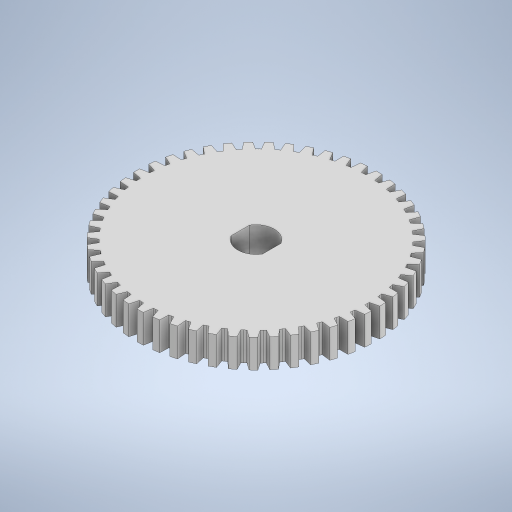
# Autodesk Inventor part: Tandwiel
Saved by Autodesk Inventor 2023.2 (Build 272271030, 271C)
## iProperties
Created: 2023-03-15
Part Number: Tandwiel
Material: Generic
Document SubType Name: Modeling
Designer: daanj
Density: 1 g/cm^3
Appearance: Default
Author: daanj
Autodesk Inventor part; units mm, degrees
ref_plane "YZ Plane" through (0, 0, 0) normal (1, 0, 0) x (0, 1, 0)
ref_plane "XZ Plane" through (0, 0, 0) normal (0, 1, 0) x (-1, 0, 0)
ref_plane "XY Plane" through (0, 0, 0) normal (0, 0, 1) x (1, 0, 0)
sketch "Sketch1" plane through (0, 0, 0) normal (0, 1, 0) x (-1, 0, 0)
  line L0 (0, 0) -> (25.1689, -1.5524) construction
  line L1 (0, 0) -> (25.1122, 1.5489) construction
  line L2 (0, 0) -> (25.4925, 0) construction
  line L3 (19.4825, 0.8259) -> (20.993, 0.5434)
  line L4 (20.993, -0.5434) -> (19.4825, -0.8259)
  line L5 (19.463, 1.2004) -> (19.4825, 0.8259)
  line L6 (19.4825, -0.8259) -> (19.463, -1.2004)
  arc A0 (20.993, -0.5434) -> (20.993, 0.5434) centre (0, 0) ccw
  line L7 (19.168, 3.5831) -> (19.2333, 3.2138)
  line L8 (19.2333, 3.2138) -> (20.7671, 3.119)
  arc A1 (20.9006, 2.0405) -> (20.7671, 3.119) centre (0, 0) ccw
  line L9 (20.9006, 2.0405) -> (19.4363, 1.5745)
  line L10 (19.4363, 1.5745) -> (19.463, 1.2004)
  line L11 (18.5824, 5.9115) -> (18.6926, 5.553)
  line L12 (18.6926, 5.553) -> (20.2264, 5.6474)
  arc A2 (20.4915, 4.5935) -> (20.2264, 5.6474) centre (0, 0) ccw
  line L13 (20.4915, 4.5935) -> (19.0955, 3.9511)
  line L14 (19.0955, 3.9511) -> (19.168, 3.5831)
  line L15 (17.7151, 8.1502) -> (17.8685, 7.808)
  line L16 (17.8685, 7.808) -> (19.3791, 8.0902)
  arc A3 (19.7717, 7.0769) -> (19.3791, 8.0902) centre (0, 0) ccw
  line L17 (19.7717, 7.0769) -> (18.4653, 6.2677)
  line L18 (18.4653, 6.2677) -> (18.5824, 5.9115)
  line L19 (16.5792, 10.2654) -> (16.7736, 9.9447)
  line L20 (16.7736, 9.9447) -> (18.238, 10.4104)
  arc A4 (18.7521, 9.4529) -> (18.238, 10.4104) centre (0, 0) ccw
  line L21 (18.7521, 9.4529) -> (17.5551, 8.4894)
  line L22 (17.5551, 8.4894) -> (17.7151, 8.1502)
  line L23 (15.1921, 12.225) -> (15.4244, 11.9306)
  line L24 (15.4244, 11.9306) -> (16.8204, 12.5727)
  arc A5 (17.4483, 11.6857) -> (16.8204, 12.5727) centre (0, 0) ccw
  line L25 (17.4483, 11.6857) -> (16.3788, 10.5824)
  line L26 (16.3788, 10.5824) -> (16.5792, 10.2654)
  line L27 (13.5746, 13.9993) -> (13.8413, 13.7356)
  line L28 (13.8413, 13.7356) -> (15.1479, 14.5444)
  arc A6 (15.8801, 13.7413) -> (15.1479, 14.5444) centre (0, 0) ccw
  line L29 (15.8801, 13.7413) -> (14.9542, 12.5149)
  line L30 (14.9542, 12.5149) -> (15.1921, 12.225)
  line L31 (11.7514, 15.5613) -> (12.0485, 15.3325)
  line L32 (12.0485, 15.3325) -> (13.2458, 16.2957)
  arc A7 (14.0711, 15.5886) -> (13.2458, 16.2957) centre (0, 0) ccw
  line L33 (14.0711, 15.5886) -> (13.3029, 14.2577)
  line L34 (13.3029, 14.2577) -> (13.5746, 13.9993)
  line L35 (9.75, 16.8875) -> (10.073, 16.6969)
  line L36 (10.073, 16.6969) -> (11.1428, 17.7999)
  arc A8 (12.0487, 17.1996) -> (11.1428, 17.7999) centre (0, 0) ccw
  line L37 (12.0487, 17.1996) -> (11.4499, 15.7844)
  line L38 (11.4499, 15.7844) -> (11.7514, 15.5613)
  line L39 (7.6008, 17.9577) -> (7.9448, 17.8082)
  line L40 (7.9448, 17.8082) -> (8.871, 19.0343)
  arc A9 (9.8438, 18.5499) -> (8.871, 19.0343) centre (0, 0) ccw
  line L41 (9.8438, 18.5499) -> (9.4234, 17.0719)
  line L42 (9.4234, 17.0719) -> (9.75, 16.8875)
  line L43 (5.3364, 18.7556) -> (5.6961, 18.6495)
  line L44 (5.6961, 18.6495) -> (6.4646, 19.9802)
  arc A10 (7.4896, 19.619) -> (6.4646, 19.9802) centre (0, 0) ccw
  line L45 (7.4896, 19.619) -> (7.2541, 18.1005)
  line L46 (7.2541, 18.1005) -> (7.6008, 17.9577)
  line L47 (2.9911, 19.2692) -> (3.3611, 19.2081)
  line L48 (3.3611, 19.2081) -> (3.9603, 20.6232)
  arc A11 (5.0219, 20.3907) -> (3.9603, 20.6232) centre (0, 0) ccw
  line L49 (5.0219, 20.3907) -> (4.9748, 18.8548)
  line L50 (4.9748, 18.8548) -> (5.3364, 18.7556)
  line L51 (0.6005, 19.4908) -> (0.9752, 19.4756)
  line L52 (0.9752, 19.4756) -> (1.3959, 20.9536)
  arc A12 (2.478, 20.8533) -> (1.3959, 20.9536) centre (0, 0) ccw
  line L53 (2.478, 20.8533) -> (2.62, 19.3232)
  line L54 (2.62, 19.3232) -> (2.9911, 19.2692)
  line L55 (-1.7992, 19.4168) -> (-1.4255, 19.4478)
  line L56 (-1.4255, 19.4478) -> (-1.1896, 20.9663)
  arc A13 (-0.1034, 20.9997) -> (-1.1896, 20.9663) centre (0, 0) ccw
  line L57 (-0.1034, 20.9997) -> (0.2256, 19.4987)
  line L58 (0.2256, 19.4987) -> (0.6005, 19.4908)
  line L59 (-4.1717, 19.0485) -> (-3.8046, 19.1252)
  line L60 (-3.8046, 19.1252) -> (-3.7571, 20.6612)
  arc A14 (-2.6832, 20.8279) -> (-3.7571, 20.6612) centre (0, 0) ccw
  line L61 (-2.6832, 20.8279) -> (-2.1723, 19.3786)
  line L62 (-2.1723, 19.3786) -> (-1.7992, 19.4168)
  line L63 (-6.4809, 18.3915) -> (-6.126, 18.5127)
  line L64 (-6.126, 18.5127) -> (-6.2676, 20.0429)
  arc A15 (-5.2224, 20.3403) -> (-6.2676, 20.0429) centre (0, 0) ccw
  line L65 (-5.2224, 20.3403) -> (-4.5372, 18.9648)
  line L66 (-4.5372, 18.9648) -> (-4.1717, 19.0485)
  line L67 (-8.6919, 17.4557) -> (-8.3546, 17.6196)
  line L68 (-8.3546, 17.6196) -> (-8.6832, 19.1207)
  arc A16 (-7.6824, 19.5443) -> (-8.6832, 19.1207) centre (0, 0) ccw
  line L69 (-7.6824, 19.5443) -> (-6.8334, 18.2635)
  line L70 (-6.8334, 18.2635) -> (-6.4809, 18.3915)
  line L71 (-10.7711, 16.2552) -> (-10.4565, 16.4594)
  line L72 (-10.4565, 16.4594) -> (-10.9671, 17.9088)
  arc A17 (-10.0259, 18.4521) -> (-10.9671, 17.9088) centre (0, 0) ccw
  line L73 (-10.0259, 18.4521) -> (-9.026, 17.2853)
  line L74 (-9.026, 17.2853) -> (-8.6919, 17.4557)
  line L75 (-12.6871, 14.8084) -> (-12.3999, 15.0496)
  line L76 (-12.3999, 15.0496) -> (-13.0847, 16.4253)
  arc A18 (-12.2175, 17.0802) -> (-13.0847, 16.4253) centre (0, 0) ccw
  line L77 (-12.2175, 17.0802) -> (-11.0817, 16.0451)
  line L78 (-11.0817, 16.0451) -> (-10.7711, 16.2552)
  line L79 (-14.4107, 13.1371) -> (-14.1554, 13.4118)
  line L80 (-14.1554, 13.4118) -> (-15.004, 14.6928)
  arc A19 (-14.2238, 15.4494) -> (-15.004, 14.6928) centre (0, 0) ccw
  line L81 (-14.2238, 15.4494) -> (-12.9695, 14.5617)
  line L82 (-12.9695, 14.5617) -> (-12.6871, 14.8084)
  line L83 (-15.9158, 11.2666) -> (-15.6962, 11.5706)
  line L84 (-15.6962, 11.5706) -> (-16.6959, 12.7377)
  arc A20 (-16.0146, 13.5843) -> (-16.6959, 12.7377) centre (0, 0) ccw
  line L85 (-16.0146, 13.5843) -> (-14.6606, 12.8575)
  line L86 (-14.6606, 12.8575) -> (-14.4107, 13.1371)
  line L87 (-17.1797, 9.2253) -> (-16.9992, 9.554)
  line L88 (-16.9992, 9.554) -> (-18.1346, 10.5894)
  arc A21 (-17.5625, 11.5134) -> (-18.1346, 10.5894) centre (0, 0) ccw
  line L89 (-17.5625, 11.5134) -> (-16.1296, 10.9584)
  line L90 (-16.1296, 10.9584) -> (-15.9158, 11.2666)
  line L91 (-18.1832, 7.0442) -> (-18.0444, 7.3926)
  line L92 (-18.0444, 7.3926) -> (-19.2985, 8.2806)
  arc A22 (-18.8443, 9.2679) -> (-19.2985, 8.2806) centre (0, 0) ccw
  line L93 (-18.8443, 9.2679) -> (-17.354, 8.8932)
  line L94 (-17.354, 8.8932) -> (-17.1797, 9.2253)
  line L95 (-18.911, 4.7563) -> (-18.8161, 5.1191)
  line L96 (-18.8161, 5.1191) -> (-20.1698, 5.8463)
  arc A23 (-19.8404, 6.8819) -> (-20.1698, 5.8463) centre (0, 0) ccw
  line L97 (-19.8404, 6.8819) -> (-18.3153, 6.6932)
  line L98 (-18.3153, 6.6932) -> (-18.1832, 7.0442)
  line L99 (-19.3522, 2.3963) -> (-19.3025, 2.768)
  line L100 (-19.3025, 2.768) -> (-20.7354, 3.3233)
  arc A24 (-20.5357, 4.3916) -> (-20.7354, 3.3233) centre (0, 0) ccw
  line L101 (-20.5357, 4.3916) -> (-18.999, 4.3918)
  line L102 (-18.999, 4.3918) -> (-18.911, 4.7563)
  line L103 (-19.5, 0) -> (-19.4964, 0.375)
  line L104 (-19.4964, 0.375) -> (-20.9866, 0.75)
  arc A25 (-20.9197, 1.8347) -> (-20.9866, 0.75) centre (0, 0) ccw
  line L105 (-20.9197, 1.8347) -> (-19.3947, 2.0237)
  line L106 (-19.3947, 2.0237) -> (-19.3522, 2.3963)
  line L107 (-19.3522, -2.3963) -> (-19.3947, -2.0237)
  line L108 (-19.3947, -2.0237) -> (-20.9197, -1.8347)
  arc A26 (-20.9866, -0.75) -> (-20.9197, -1.8347) centre (0, 0) ccw
  line L109 (-20.9866, -0.75) -> (-19.4964, -0.375)
  line L110 (-19.4964, -0.375) -> (-19.5, 0)
  line L111 (-18.911, -4.7563) -> (-18.999, -4.3918)
  line L112 (-18.999, -4.3918) -> (-20.5357, -4.3916)
  arc A27 (-20.7354, -3.3233) -> (-20.5357, -4.3916) centre (0, 0) ccw
  line L113 (-20.7354, -3.3233) -> (-19.3025, -2.768)
  line L114 (-19.3025, -2.768) -> (-19.3522, -2.3963)
  line L115 (-18.1832, -7.0442) -> (-18.3153, -6.6932)
  line L116 (-18.3153, -6.6932) -> (-19.8404, -6.8819)
  arc A28 (-20.1698, -5.8463) -> (-19.8404, -6.8819) centre (0, 0) ccw
  line L117 (-20.1698, -5.8463) -> (-18.8161, -5.1191)
  line L118 (-18.8161, -5.1191) -> (-18.911, -4.7563)
  line L119 (-17.1797, -9.2253) -> (-17.354, -8.8932)
  line L120 (-17.354, -8.8932) -> (-18.8443, -9.2679)
  arc A29 (-19.2985, -8.2806) -> (-18.8443, -9.2679) centre (0, 0) ccw
  line L121 (-19.2985, -8.2806) -> (-18.0444, -7.3926)
  line L122 (-18.0444, -7.3926) -> (-18.1832, -7.0442)
  line L123 (-15.9158, -11.2666) -> (-16.1296, -10.9584)
  line L124 (-16.1296, -10.9584) -> (-17.5625, -11.5134)
  arc A30 (-18.1346, -10.5894) -> (-17.5625, -11.5134) centre (0, 0) ccw
  line L125 (-18.1346, -10.5894) -> (-16.9992, -9.554)
  line L126 (-16.9992, -9.554) -> (-17.1797, -9.2253)
  line L127 (-14.4107, -13.1371) -> (-14.6606, -12.8575)
  line L128 (-14.6606, -12.8575) -> (-16.0146, -13.5843)
  arc A31 (-16.6959, -12.7377) -> (-16.0146, -13.5843) centre (0, 0) ccw
  line L129 (-16.6959, -12.7377) -> (-15.6962, -11.5706)
  line L130 (-15.6962, -11.5706) -> (-15.9158, -11.2666)
  line L131 (-12.6871, -14.8084) -> (-12.9695, -14.5617)
  line L132 (-12.9695, -14.5617) -> (-14.2238, -15.4494)
  arc A32 (-15.004, -14.6928) -> (-14.2238, -15.4494) centre (0, 0) ccw
  line L133 (-15.004, -14.6928) -> (-14.1554, -13.4118)
  line L134 (-14.1554, -13.4118) -> (-14.4107, -13.1371)
  line L135 (-10.7711, -16.2552) -> (-11.0817, -16.0451)
  line L136 (-11.0817, -16.0451) -> (-12.2175, -17.0802)
  arc A33 (-13.0847, -16.4253) -> (-12.2175, -17.0802) centre (0, 0) ccw
  line L137 (-13.0847, -16.4253) -> (-12.3999, -15.0496)
  line L138 (-12.3999, -15.0496) -> (-12.6871, -14.8084)
  line L139 (-8.6919, -17.4557) -> (-9.026, -17.2853)
  line L140 (-9.026, -17.2853) -> (-10.0259, -18.4521)
  arc A34 (-10.9671, -17.9088) -> (-10.0259, -18.4521) centre (0, 0) ccw
  line L141 (-10.9671, -17.9088) -> (-10.4565, -16.4594)
  line L142 (-10.4565, -16.4594) -> (-10.7711, -16.2552)
  line L143 (-6.4809, -18.3915) -> (-6.8334, -18.2635)
  line L144 (-6.8334, -18.2635) -> (-7.6824, -19.5443)
  arc A35 (-8.6832, -19.1207) -> (-7.6824, -19.5443) centre (0, 0) ccw
  line L145 (-8.6832, -19.1207) -> (-8.3546, -17.6196)
  line L146 (-8.3546, -17.6196) -> (-8.6919, -17.4557)
  line L147 (-4.1717, -19.0485) -> (-4.5372, -18.9648)
  line L148 (-4.5372, -18.9648) -> (-5.2224, -20.3403)
  arc A36 (-6.2676, -20.0429) -> (-5.2224, -20.3403) centre (0, 0) ccw
  line L149 (-6.2676, -20.0429) -> (-6.126, -18.5127)
  line L150 (-6.126, -18.5127) -> (-6.4809, -18.3915)
  line L151 (-1.7992, -19.4168) -> (-2.1723, -19.3786)
  line L152 (-2.1723, -19.3786) -> (-2.6832, -20.8279)
  arc A37 (-3.7571, -20.6612) -> (-2.6832, -20.8279) centre (0, 0) ccw
  line L153 (-3.7571, -20.6612) -> (-3.8046, -19.1252)
  line L154 (-3.8046, -19.1252) -> (-4.1717, -19.0485)
  line L155 (0.6005, -19.4908) -> (0.2256, -19.4987)
  line L156 (0.2256, -19.4987) -> (-0.1034, -20.9997)
  arc A38 (-1.1896, -20.9663) -> (-0.1034, -20.9997) centre (0, 0) ccw
  line L157 (-1.1896, -20.9663) -> (-1.4255, -19.4478)
  line L158 (-1.4255, -19.4478) -> (-1.7992, -19.4168)
  line L159 (2.9911, -19.2692) -> (2.62, -19.3232)
  line L160 (2.62, -19.3232) -> (2.478, -20.8533)
  arc A39 (1.3959, -20.9536) -> (2.478, -20.8533) centre (0, 0) ccw
  line L161 (1.3959, -20.9536) -> (0.9752, -19.4756)
  line L162 (0.9752, -19.4756) -> (0.6005, -19.4908)
  line L163 (5.3364, -18.7556) -> (4.9748, -18.8548)
  line L164 (4.9748, -18.8548) -> (5.0219, -20.3907)
  arc A40 (3.9603, -20.6232) -> (5.0219, -20.3907) centre (0, 0) ccw
  line L165 (3.9603, -20.6232) -> (3.3611, -19.2081)
  line L166 (3.3611, -19.2081) -> (2.9911, -19.2692)
  line L167 (7.6008, -17.9577) -> (7.2541, -18.1005)
  line L168 (7.2541, -18.1005) -> (7.4896, -19.619)
  arc A41 (6.4646, -19.9802) -> (7.4896, -19.619) centre (0, 0) ccw
  line L169 (6.4646, -19.9802) -> (5.6961, -18.6495)
  line L170 (5.6961, -18.6495) -> (5.3364, -18.7556)
  line L171 (9.75, -16.8875) -> (9.4234, -17.0719)
  line L172 (9.4234, -17.0719) -> (9.8438, -18.5499)
  arc A42 (8.871, -19.0343) -> (9.8438, -18.5499) centre (0, 0) ccw
  line L173 (8.871, -19.0343) -> (7.9448, -17.8082)
  line L174 (7.9448, -17.8082) -> (7.6008, -17.9577)
  line L175 (11.7514, -15.5613) -> (11.4499, -15.7844)
  line L176 (11.4499, -15.7844) -> (12.0487, -17.1996)
  arc A43 (11.1428, -17.7999) -> (12.0487, -17.1996) centre (0, 0) ccw
  line L177 (11.1428, -17.7999) -> (10.073, -16.6969)
  line L178 (10.073, -16.6969) -> (9.75, -16.8875)
  line L179 (13.5746, -13.9993) -> (13.3029, -14.2577)
  line L180 (13.3029, -14.2577) -> (14.0711, -15.5886)
  arc A44 (13.2458, -16.2957) -> (14.0711, -15.5886) centre (0, 0) ccw
  line L181 (13.2458, -16.2957) -> (12.0485, -15.3325)
  line L182 (12.0485, -15.3325) -> (11.7514, -15.5613)
  line L183 (15.1921, -12.225) -> (14.9542, -12.5149)
  line L184 (14.9542, -12.5149) -> (15.8801, -13.7413)
  arc A45 (15.1479, -14.5444) -> (15.8801, -13.7413) centre (0, 0) ccw
  line L185 (15.1479, -14.5444) -> (13.8413, -13.7356)
  line L186 (13.8413, -13.7356) -> (13.5746, -13.9993)
  line L187 (16.5792, -10.2654) -> (16.3788, -10.5824)
  line L188 (16.3788, -10.5824) -> (17.4483, -11.6857)
  arc A46 (16.8204, -12.5727) -> (17.4483, -11.6857) centre (0, 0) ccw
  line L189 (16.8204, -12.5727) -> (15.4244, -11.9306)
  line L190 (15.4244, -11.9306) -> (15.1921, -12.225)
  line L191 (17.7151, -8.1502) -> (17.5551, -8.4894)
  line L192 (17.5551, -8.4894) -> (18.7521, -9.4529)
  arc A47 (18.238, -10.4104) -> (18.7521, -9.4529) centre (0, 0) ccw
  line L193 (18.238, -10.4104) -> (16.7736, -9.9447)
  line L194 (16.7736, -9.9447) -> (16.5792, -10.2654)
  line L195 (18.5824, -5.9115) -> (18.4653, -6.2677)
  line L196 (18.4653, -6.2677) -> (19.7717, -7.0769)
  arc A48 (19.3791, -8.0902) -> (19.7717, -7.0769) centre (0, 0) ccw
  line L197 (19.3791, -8.0902) -> (17.8685, -7.808)
  line L198 (17.8685, -7.808) -> (17.7151, -8.1502)
  line L199 (19.168, -3.5831) -> (19.0955, -3.9511)
  line L200 (19.0955, -3.9511) -> (20.4915, -4.5935)
  arc A49 (20.2264, -5.6474) -> (20.4915, -4.5935) centre (0, 0) ccw
  line L201 (20.2264, -5.6474) -> (18.6926, -5.553)
  line L202 (18.6926, -5.553) -> (18.5824, -5.9115)
  line L203 (19.463, -1.2004) -> (19.4363, -1.5745)
  line L204 (19.4363, -1.5745) -> (20.9006, -2.0405)
  arc A50 (20.7671, -3.119) -> (20.9006, -2.0405) centre (0, 0) ccw
  line L205 (20.7671, -3.119) -> (19.2333, -3.2138)
  line L206 (19.2333, -3.2138) -> (19.168, -3.5831)
  dimension "d1" = 7.059
  dimension "d2" = 3.529
  dimension "d4" = 0.375
  dimension "d5" = 0.375
  dimension "d7" = 0.75
  dimension "d8" = 0.75
  dimension "d9" = 1.0868
  dimension "d12" = 360
  constraints: 414 end point, 102 point on circle, 51 centre point, 2 point on line, 1 coincident, 1 horizontal, 613 other
  measures "d1" angle of L0 L1
  measures "d2" angle of L2 L0
  measures "d4" distance from line of L3.start L1
  measures "d5" distance from line of L0 L4.end
  measures "d7" distance from line of L1 L3.end
  measures "d8" distance from line of L0 L4.start
  measures "d9" distance of L3.end L4.start
extrude "Extrusion1" add sketch "Sketch1" along normal blind 5
sketch "Sketch4" plane through (0, 5, 0) normal (0, 1, 0) x (1, 0, 0)
  line L0 (2.7713, 1.6) -> (2.7713, -1.6)
  line L1 (-2.7713, 1.6) -> (-2.7713, -1.6)
  arc A0 (-2.7713, -1.6) -> (2.7713, -1.6) centre (0, 0) ccw
  arc A1 (2.7713, 1.6) -> (-2.7713, 1.6) centre (0, 0) ccw
  dimension "d27" = 3.2
  dimension "d28" = 3.2
  constraints: 4 end point, 4 point on circle, 2 centre point, 1 coincident, 1 parallel, 1 vertical
  measures "d27" distance of L1.start L1.end
  measures "d28" distance of L0.start L0.end
extrude "Extrusion4" cut sketch "Sketch4" along normal mid plane 10
body "Solid1"
